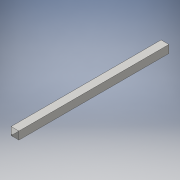
# Autodesk Inventor part: Pin
Saved by Autodesk Inventor 2016 (Build 200138000, 138)
## iProperties
Created: 2016-04-16
Part Number: Pin
Material: Generic
Document SubType Name: Modeling
Designer: Jarrett
Density: 1 g/cm^3
Appearance: Default
Author: Jarrett
Autodesk Inventor part; units mm, degrees
ref_plane "YZ Plane" through (0, 0, 0) normal (1, 0, 0) x (0, 1, 0)
ref_plane "XZ Plane" through (0, 0, 0) normal (0, 1, 0) x (-1, 0, 0)
ref_plane "XY Plane" through (0, 0, 0) normal (0, 0, 1) x (1, 0, 0)
sketch "Sketch1" plane through (0, 0, 0) normal (0, 1, 0) x (-1, 0, 0)
  line L0 (0, 0) -> (0.6, 0)
  line L1 (0.6, 0) -> (0.6, -0.6)
  line L2 (0.6, -0.6) -> (0, -0.6)
  line L3 (0, -0.6) -> (0, 0)
  dimension "d0" = 0.6
  constraints: 8 end point, 2 parallel, 2 perpendicular, 1 horizontal
  measures "d0" distance of L0.end L1.end
extrude "Extrusion1" add sketch "Sketch1" along normal blind 12
chamfer "Chamfer1" distance 0.25 angle 45 8 edges at (0, 12, -0.3) (-0.3, 12, 0) (-0.6, 12, -0.3) (-0.3, 12, -0.6) (-0.6, 0, -0.3) (-0.3, 0, -0.6) (0, 0, -0.3) (-0.3, 0, 0)
body "Solid1"
